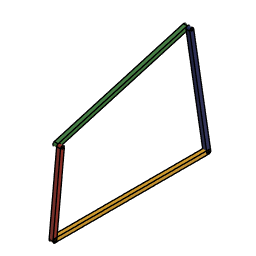
Crank Rocker v1 (Autodesk Fusion 360 design; units mm, degrees)
Autodesk Fusion 360 part; units mm, degrees
sketch "Sketch1" plane through (0, 0, 0) normal (1, 0, 0) x (0, 1, 0)
  line L0 (20, -0.5) -> (-20, -0.5)
  line L1 (-20, 0.5) -> (20, 0.5)
  line L2 (20, -0.5) -> (-20, 0.5) construction
  line L3 (-20, -0.5) -> (20, 0.5) construction
  arc A0 (-19.975, 0.4994) -> (-19.975, -0.4994) centre (-20, 0) ccw
  arc A1 (19.975, -0.4994) -> (19.975, 0.4994) centre (20, 0) ccw
  circle A2 centre (-20, 0) radius 0.25
  circle A3 centre (20, 0) radius 0.25
  dimension "d1" = 40
  dimension "d2" = 0.5
  dimension "d3" = 0.5
  constraint horizontal L0
  constraint parallel L0 L1
  constraint coincident L2 origin
  constraint coincident L3 origin
  constraint coincident L0.end A0
  constraint tangent L0 A0
  constraint coincident L1.start A0
  constraint coincident L0.start A1
  constraint tangent L0 A1
  constraint coincident L1.end A1
  constraint coincident L0 A0.end
  constraint coincident L1 A0.start
  constraint coincident L1 A1.end
  constraint coincident L0 A1.start
  measures "d1" distance of L1.start L1.end
  measures "d2" diameter of A2
  measures "d3" diameter of A3
extrude "Extrude1" add sketch "Sketch1" along normal blind 1 makes body 1
sketch "Sketch2" plane through (0, 0, 0) normal (1, 0, 0) x (0, 1, 0)
  line L0 (10, -0.5) -> (-10, -0.5)
  line L1 (-10, 0.5) -> (10, 0.5)
  line L2 (10, -0.5) -> (-10, 0.5) construction
  line L3 (-10, -0.5) -> (10, 0.5) construction
  arc A0 (-9.9501, 0.4975) -> (-9.9501, -0.4975) centre (-10, 0) ccw
  arc A1 (9.9501, -0.4975) -> (9.9501, 0.4975) centre (10, 0) ccw
  circle A2 centre (-10, 0) radius 0.25
  circle A3 centre (10, 0) radius 0.25
  dimension "d6" = 20
  dimension "d7" = 0.5
  dimension "d8" = 0.5
  constraint horizontal L0
  constraint parallel L0 L1
  constraint coincident L2 origin
  constraint coincident L3 origin
  constraint coincident L0.end A0
  constraint coincident L1.start A0
  constraint coincident L0.start A1
  constraint tangent L0 A1
  constraint coincident L1.end A1
  constraint coincident L3 A0.end
  constraint coincident L2 A0.start
  constraint coincident L3 A1.end
  constraint coincident L2 A1.start
  constraint concentric A0 A2
  constraint concentric A1 A3
  measures "d6" distance of L1.start L1.end
  measures "d7" diameter of A2
  measures "d8" diameter of A3
extrude "Extrude2" add sketch "Sketch2" along normal blind 1 separate body makes body 2
sketch "Sketch3" plane through (0, 0, 0) normal (1, 0, 0) x (0, 1, 0)
  line L0 (17.5, -0.5) -> (-17.5, -0.5)
  line L1 (-17.5, 0.5) -> (17.5, 0.5)
  line L2 (17.5, -0.5) -> (-17.5, 0.5) construction
  line L3 (-17.5, -0.5) -> (17.5, 0.5) construction
  arc A0 (-17.4715, 0.4992) -> (-17.4715, -0.4992) centre (-17.5, 0) ccw
  arc A1 (17.4715, -0.4992) -> (17.4715, 0.4992) centre (17.5, 0) ccw
  circle A2 centre (-17.5, 0) radius 0.25
  circle A3 centre (17.5, 0) radius 0.25
  dimension "d11" = 35
  dimension "d12" = 0.5
  dimension "d13" = 0.5
  constraint horizontal L0
  constraint parallel L0 L1
  constraint coincident L2 origin
  constraint coincident L3 origin
  constraint coincident L0.end A0
  constraint coincident L1.start A0
  constraint coincident L0.start A1
  constraint tangent L0 A1
  constraint coincident L1.end A1
  constraint coincident L0 A0.end
  constraint coincident L1 A0.start
  constraint coincident L1 A1.end
  constraint coincident L0 A1.start
  measures "d11" distance of L1.start L1.end
  measures "d12" diameter of A2
  measures "d13" diameter of A3
extrude "Extrude3" add sketch "Sketch3" along normal blind 1 separate body makes body 3
sketch "Sketch4" plane through (0, 0, 0) normal (1, 0, 0) x (0, 1, 0)
  line L0 (15, -0.5) -> (-15, -0.5)
  line L1 (-15, 0.5) -> (15, 0.5)
  line L2 (15, -0.5) -> (-15, 0.5) construction
  line L3 (-15, -0.5) -> (15, 0.5) construction
  arc A0 (-14.9667, 0.4989) -> (-14.9667, -0.4989) centre (-15, 0) ccw
  arc A1 (14.9667, -0.4989) -> (14.9667, 0.4989) centre (15, 0) ccw
  circle A2 centre (-15, 0) radius 0.25
  circle A3 centre (15, 0) radius 0.25
  dimension "d16" = 30
  dimension "d17" = 0.5
  dimension "d18" = 0.5
  constraint horizontal L0
  constraint parallel L0 L1
  constraint coincident L2 origin
  constraint coincident L3 origin
  constraint coincident L0.end A0
  constraint tangent L0 A0
  constraint coincident L1.start A0
  constraint coincident L0.start A1
  constraint tangent L0 A1
  constraint coincident L1.end A1
  constraint coincident L3 A0.end
  constraint coincident L2 A0.start
  constraint coincident L3 A1.end
  constraint coincident L2 A1.start
  constraint concentric A0 A2
  constraint concentric A1 A3
  measures "d16" distance of L1.start L1.end
  measures "d17" diameter of A2
  measures "d18" diameter of A3
extrude "Extrude4" add sketch "Sketch4" along normal blind 1 separate body makes body 4
copy_body "Body->Comp1" bodies 4 removing the originals makes body 5 in component "3cmL4"
copy_body "Body->Comp2" bodies 3 removing the originals makes body 6 in component "3.5cmL3"
copy_body "Body->Comp3" bodies 2 removing the originals makes body 7 in component "2cmL2"
copy_body "Body->Comp4" bodies 1 removing the originals makes body 8 in component "4cmL1"
component "3cmL4" placed x (-1, 0, 0) y (0, -0.364583, -0.931171) z (0, -0.931171, 0.364583) at (1, 14.5312, -13.9676)
component "3.5cmL3" placed x (1, 0, 0) y (0, 0.282145, -0.959372) z (0, 0.959372, 0.282145) at (-1, 4.125, -11.1461)
component "2cmL2" placed x (-1, 0, 0) y (0, 0.959372, 0.282145) z (0, 0.282145, -0.959372) at (1, -10.4063, 2.8214)
component "4cmL1" placed x (1, 0, 0) y (0, 1, 0) z (0, 0, 1) at (0, 0, 0)
named bodies: "4cmL1", "2cmL2", "3.5cmL3", "3cmL4"
